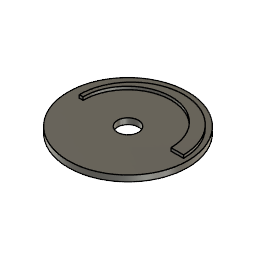
Armrest - Front section L and R (Autodesk Fusion 360 archive; units mm, degrees)
design "poten dial"
Autodesk Fusion 360 part; units mm, degrees
sketch "Sketch1" plane through (0, 0, 0) normal (0, 0, 1) x (1, 0, 0)
  circle A0 centre (0, 0) radius 20
  circle A1 centre (0, 0) radius 3.5
  dimension "d1" = 40
  dimension "d11" = 7
  constraint coincident A0.centre A1.centre
  constraint concentric A0 A1
  measures "d1" diameter of A0
  measures "d11" diameter of A1
extrude "Extrude1" add sketch "Sketch1" along normal blind 2 makes body 1
sketch "Sketch2" plane through (0, 0, 2) normal (0, 0, 1) x (-1, 0, 0)
  circle A0 centre (0, 0) radius 20
  circle A1 centre (0, 0) radius 3.5
  circle A2 centre (0, 0) radius 12.5
  ellipse E0 centre (-1.1293, 0) end of major axis (16.3342, 0) minor radius 17.5145
  line L0 (-18.5928, 0) -> (16.3342, 0) construction
  line L1 (-1.1293, -17.5145) -> (-1.1293, 17.5145) construction
  ellipse E1 centre (0.3342, 0) end of major axis (15.0661, 0) minor radius 14.7954
  line L2 (-14.3977, 0) -> (15.0661, 0) construction
  line L3 (0.3342, -14.7954) -> (0.3342, 14.7954) construction
  line L4 (0, 0) -> (20, 0)
  line L5 (0, 0) -> (-20, 0)
  line L6 (-1.1293, 0) -> (0.3342, 0)
  dimension "d16" = 25
  constraint concentric A0 A2
  constraint coincident E0 L0.start
  constraint coincident E0 L0.end
  constraint coincident E0 L1.start
  constraint coincident E0 L1.end
  constraint horizontal L0
  constraint coincident E1 L2.start
  constraint coincident E1 L2.end
  constraint coincident E1 L3.start
  constraint coincident E1 L3.end
  constraint coincident L0 E1.centre
  constraint perpendicular L1 L2
  constraint coincident A0.centre A1.centre
  constraint coincident A0 L4.end
  constraint parallel L0 L4
  constraint coincident A0 L5.end
  constraint parallel L4 L5
  constraint coincident L0 E0.centre
  constraint coincident E1.centre L6.end
  constraint coincident E0.centre L6.start
  constraint coincident L0.start L5
  measures "d16" diameter of A2
extrude "Extrude3" cut sketch "Sketch2" against normal blind 3 contours E0 E1 L4 L5 picked at (-16.786, -3.5333) bodies 1
extrude "Extrude2" add sketch "Sketch2" along normal blind 3 from surface at -2 separate body contours E0 E1 L4 L5 picked at (-16.786, -3.5333) makes body 2

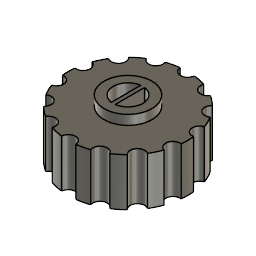
design "potentiometer knob"
Autodesk Fusion 360 part; units mm, degrees
sketch "Sketch1" plane through (0, 0, 0) normal (0, 0, 1) x (1, 0, 0)
  circle A0 centre (0, 0) radius 3.1
  line L0 (-0.4, 3.1) -> (0.4, 3.1)
  line L1 (0.4, 3.1) -> (0.4, -3.1)
  line L2 (0.4, -3.1) -> (-0.4, -3.1)
  line L3 (-0.4, -3.1) -> (-0.4, 3.1)
  line L4 (0, 0) -> (0, 3.1)
  circle A1 centre (0, 0) radius 5
  dimension "d1" = 6.2
  dimension "d2" = 0.8
  dimension "d3" = 6.2
  dimension "d4" = 10
  constraint coincident A0.centre L4.start
  constraint horizontal L0
  constraint vertical L1
  constraint horizontal L2
  constraint vertical L3
  constraint coincident A0 L4.end
  constraint parallel L3 L4
  constraint midpoint L0 L4.end
  measures "d1" diameter of A0
  measures "d2" distance of L0.start L0.end
  measures "d3" distance of L0.start L2.end
  measures "d4" diameter of A1
extrude "Extrude1" add sketch "Sketch1" along normal blind 7 contours A0 L1 L3 | A0 L0 L1 | A0 L1 L2 | A0 L0 L3 | A0 L2 L3 | A1
sketch "Sketch2" plane through (0, 0, 0) normal (0, 0, 1) x (1, 0, 0)
  circle A0 centre (0, 0) radius 12.5
  circle A1 centre (0, -12.5) radius 1.5
  circle A2 centre (5.4235, -11.2621) radius 1.5
  circle A3 centre (9.7729, -7.7936) radius 1.5
  circle A4 centre (12.1866, -2.7815) radius 1.5
  circle A5 centre (12.1866, 2.7815) radius 1.5
  circle A6 centre (9.7729, 7.7936) radius 1.5
  circle A7 centre (5.4235, 11.2621) radius 1.5
  circle A8 centre (0, 12.5) radius 1.5
  circle A9 centre (-5.4235, 11.2621) radius 1.5
  circle A10 centre (-9.7729, 7.7936) radius 1.5
  circle A11 centre (-12.1866, 2.7815) radius 1.5
  circle A12 centre (-12.1866, -2.7815) radius 1.5
  circle A13 centre (-9.7729, -7.7936) radius 1.5
  circle A14 centre (-5.4235, -11.2621) radius 1.5
  circle A15 centre (0, 0) radius 5
  line L0 (12.5, 0.6) -> (5.5, 0.6)
  line L1 (5.5, 0.6) -> (5.5, -0.6)
  line L2 (5.5, -0.6) -> (12.5, -0.6)
  line L3 (12.5, -0.6) -> (12.5, 0.6)
  line L4 (0, 0) -> (12.5, 0)
  dimension "d7" = 25
  dimension "d8" = 3
  dimension "d10" = 360
  dimension "d13" = 10
  dimension "d16" = 7
  dimension "d17" = 1.2
  constraint coincident A0.centre A15.centre
  constraint coincident A0 A1.centre
  constraint horizontal L0
  constraint vertical L1
  constraint horizontal L2
  constraint vertical L3
  constraint coincident A0 L4.end
  constraint horizontal L4
  constraint midpoint L3 L4.end
  measures "d7" diameter of A0
  measures "d8" diameter of A1
  measures "d13" diameter of A15
  measures "d16" distance of L0.start L0.end
  measures "d17" distance of L0.start L2.end
extrude "Extrude2" add sketch "Sketch2" against normal blind 5 contours A0 L0 L1 L4 | A0 L1 L2 L4 | A0 A1 A2 A3 A4 A5 A6 A7 A8 A9 A10 A11 A12 A13 A14 L0 L1 L2 | A15
extrude "Extrude3" add sketch "Sketch2" along normal blind 5 contours A0 L0 L1 L4 | A0 L1 L2 L4 | A0 A1 A2 A3 A4 A5 A6 A7 A8 A9 A10 A11 A12 A13 A14 L0 L1 L2
